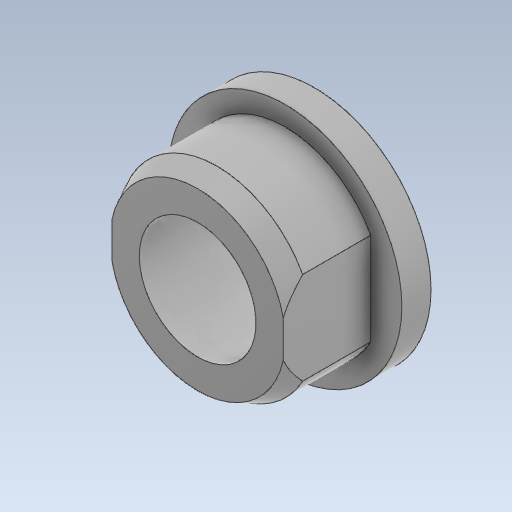
# Autodesk Inventor part: LED-0606
Saved by Autodesk Inventor 2020 (Build 240168000, 168)
## iProperties
Created: 2021-10-14
Part Number: LED-0606
Material: アセタール樹脂、黒
Document SubType Name: Modeling
Designer: Masato Kubotera
Density: 1.425 g/cm^3
Appearance: 滑らか - 標準の灰色
Description: 既製品
Mass: 0.471056 g
Surface Area: 4.68851 cm^2
Volume: 0.330566 cm^3
Catalog Web Link: https://jp.misumi-ec.com/vona2/detail/221000090992/?PNSearch=LED-0606&HissuCode=LED-0606&searchFlow=preview2products&Keyword=LED-0606&list=SuggestPreview
Author: Masato Kubotera
Autodesk Inventor part; units mm, degrees
ref_plane "YZ Plane" through (0, 0, 0) normal (1, 0, 0) x (0, 1, 0)
ref_plane "XZ Plane" through (0, 0, 0) normal (0, 1, 0) x (-1, 0, 0)
ref_plane "XY Plane" through (0, 0, 0) normal (0, 0, 1) x (1, 0, 0)
sketch "スケッチ1" plane through (0, 0, 0) normal (0, 1, 0) x (-1, 0, 0)
  line L0 (3, 0) -> (6, 0)
  line L1 (6, 0) -> (6, 1.5)
  line L2 (6, 1.5) -> (5, 1.5)
  line L3 (5, 1.5) -> (5, 5)
  line L4 (4.5, 6) -> (3, 6)
  line L5 (3, 6) -> (3, 6)
  line L6 (0, 6) -> (0, 0) construction
  line L7 (3, 6) -> (3, 0)
  line L8 (5, 5) -> (4.5, 6)
  dimension "d0" = 3
  dimension "d4" = 6
  dimension "d5" = 1.5
  dimension "d6" = 6
  dimension "d8" = 5
  dimension "d9" = 1
  dimension "d10" = 0.5
  constraints: 18 end point, 5 perpendicular, 2 parallel, 2 point on line, 1 horizontal
  measures "d0" distance of L6.start L5.end
  measures "d4" distance of L6.end L6.start
  measures "d5" distance of L0.end L1.end
  measures "d6" distance of L6.end L0.end
  measures "d8" horizontal distance of L3.end L6.start
  measures "d9" vertical distance of L3.end L4.start
  measures "d10" horizontal distance of L4.start L3.end
revolve "回転1" add sketch "スケッチ1" angle 360 about axis through (0, 0, 6) along (0, 0, -1)
sketch "スケッチ2" plane through (0, 0, 6) normal (0, 0, 1) x (1, 0, 0)
  line L0 (4.4, -2.3749) -> (-4.4, -2.3749)
  line L1 (-4.4, -2.3749) -> (-4.4, 2.3749)
  line L2 (-4.4, 2.3749) -> (4.4, 2.3749)
  line L3 (4.4, 2.3749) -> (4.4, -2.3749)
  line L4 (4.4, -2.3749) -> (-4.4, 2.3749) construction
  line L5 (-4.4, -2.3749) -> (4.4, 2.3749) construction
  circle A0 centre (0, 0) radius 5
  dimension "d12" = 10
  dimension "d11" = 8.8
  constraints: 12 end point, 2 midpoint, 2 parallel, 1 coincident, 1 horizontal, 1 perpendicular, 3 other
  measures "d11" distance of L1.end L2.end
extrude "押し出し1" cut sketch "スケッチ2" against normal up to surface (4.5 mm away) contours L3 A0 | A0 L1
